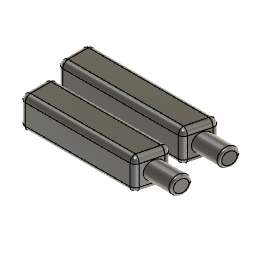
Sticks_2 v0 (Autodesk Fusion 360 design; units mm, degrees)
Autodesk Fusion 360 part; units mm, degrees
sketch "Sketch1" plane through (0, 0, 0) normal (0, 0, 1) x (1, 0, 0)
  line L0 (0, 0) -> (30, 0)
  line L1 (30, 0) -> (30, 5.8)
  line L2 (30, 5.8) -> (0, 5.8)
  line L3 (0, 5.8) -> (0, 0)
  dimension "d1" = 30
  dimension "d2" = 5.8
  constraint horizontal L0
  constraint vertical L1
  constraint horizontal L2
  constraint vertical L3
  constraint coincident L0.start L3.end
  measures "d1" distance of L0.start L0.end
  measures "d2" distance of L0.start L2.end
extrude "Extrude1" add sketch "Sketch1" along normal blind 5.8 makes body 1
sketch "Sketch2" plane through (0, 0, 0) normal (-1, 0, 0) x (0, -1, 0)
  line L0 (-5.8, 0) -> (0, 0)
  line L1 (0, 0) -> (0, 5.8)
  line L2 (0, 5.8) -> (-5.8, 5.8)
  line L3 (-5.8, 5.8) -> (-5.8, 0)
  circle A0 centre (-3, 3) radius 1.65
  dimension "d5" = 3.3
  measures "d5" diameter of A0
sketch "Sketch3" plane through (0, 0, 5.8) normal (0, 0, 1) x (-1, 0, 0)
  line L0 (0, -5.8) -> (0, 0)
  line L1 (0, 0) -> (-30, 0)
  line L2 (-30, 0) -> (-30, -5.8)
  line L3 (-30, -5.8) -> (0, -5.8)
  line L4 (-30, -5.8) -> (-28.5, 0) construction
  line L5 (-30, -5.8) -> (-24.0052, -5.8) construction
  line L6 (-30, -5.8) -> (-24.8355, -5.8)
  line L7 (-23.3355, 0) -> (-28.5, 0)
  line L8 (-23.3355, 0) -> (-24.8355, -5.8)
  line L9 (-28.5, 0) -> (-30, 0)
  line L10 (-30, -5.8) -> (-30, 0)
  dimension "d6" = 75.5
  dimension "d7" = 5
  constraint horizontal L5
  constraint coincident L2.end L3.start
  constraint coincident L1 L4.end
  constraint coincident L3 L6.end
  constraint perpendicular L2 L6
  constraint coincident L1 L7.start
  constraint parallel L1 L7
  constraint parallel L4 L8
  constraint coincident L1.end L2.start
  measures "d6" angle of L4 L5
  measures "d7" distance of L4 L8
extrude "Extrude2" cut sketch "Sketch3" against normal through all contours L1 L2 L3 L6 L7 L8 L9 L10 bodies 1
extrude "Extrude3" add sketch "Sketch2" against normal blind 30 contours A0 bodies 1
sketch "Sketch4" plane through (0, 0, 0) normal (-1, 0, 0) x (0, -1, 0)
  line L0 (-5.8, 0) -> (0, 0)
  line L1 (0, 0) -> (0, 5.8)
  line L2 (0, 5.8) -> (-5.8, 5.8)
  line L3 (-5.8, 5.8) -> (-5.8, 0)
  circle A0 centre (-2.9, 2.9) radius 1.65
  line L4 (-5.8, 5.8) -> (0, 0) construction
  dimension "d11" = 3.3
  constraint coincident L2.end L3.start
  constraint coincident L0.end L1.start
  constraint midpoint A0.centre L4
  measures "d11" diameter of A0
extrude "Extrude4" cut sketch "Sketch4" against normal blind 5 contours A0 bodies 1
sketch "Sketch5" plane through (0, 0, 5.8) normal (0, 0, 1) x (-1, 0, 0)
  line L0 (-23.3355, 0) -> (-24.8355, -5.8)
  line L1 (-24.8355, -5.8) -> (0, -5.8)
  line L2 (0, -5.8) -> (0, 0)
  line L3 (0, 0) -> (-23.3355, 0)
  line L4 (-28.5, 0) -> (-30, -5.8)
  line L5 (-30, -5.8) -> (-30, 0)
  line L6 (-30, 0) -> (-28.5, 0)
  constraint vertical L5
  constraint perpendicular L5 L6
extrude "Extrude5" cut sketch "Sketch5" against normal through all contours L4 L5 L6 bodies 1
fillet "Fillet1" radius 0.5 1 edges at (29.7026, 4.65, 3) on bodies 1
copy_body "CopyPasteBodies1" bodies 1 makes body 2
move_body "Move1" bodies 2 to x (1, 0, 0) y (0, 1, 0) z (0, 0, 1) at (0, -9, 0)
extrude "Extrude6" cut 1 faces at (0, -6.0589, 5.3818) along direction (1, 0, 0) blind 2 on bodies 2 bodies 2
extrude "Extrude7" cut 1 faces at (5, -6.5854, 3.2741) along direction (1, 0, 0) blind 2 on bodies 2 bodies 2
fillet "Fillet2" radius 1 24 edges at (12.4177, 5.8, 0) (11.6678, 0, 0) (24.8355, 5.8, 2.9) (12.4177, 5.8, 5.8) (0, 5.8, 2.9) (0, 2.9, 0) (24.0855, 2.9, 0) (23.3355, 0, 2.9) (24.0855, 2.9, 5.8) (11.6678, 0, 5.8) (0, 0, 2.9) (0, 2.9, 5.8) (12.6678, -9, 5.8) (13.4177, -3.2, 5.8) (12.6678, -9, 0) (24.0855, -6.1, 5.8) (2, -6.1, 5.8) (2, -9, 2.9) (23.3355, -9, 2.9) (24.0855, -6.1, 0) (13.4177, -3.2, 0) (2, -6.1, 0) (2, -3.2, 2.9) (24.8355, -3.2, 2.9) on bodies 1 2
chamfer "Chamfer1" distance 0.2 angle 45 2 edges at (0, 4.4383, 3.4967) (2, -4.5617, 2.3033) on bodies 1 2
